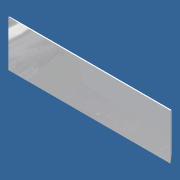
# Autodesk Inventor part: bottom panel right
Saved by Autodesk Inventor 2012 (Build 160160000, 160)
## iProperties
Created: 2012-02-06
Part Number: bottom panel right
Material: Default
Document SubType Name: Modeling
Designer: Allison Garza
Density: 1 g/cm^3
Author: Allison Garza
Autodesk Inventor part; units mm, degrees
ref_plane "YZ Plane" through (0, 0, 0) normal (1, 0, 0) x (0, 1, 0)
ref_plane "XZ Plane" through (0, 0, 0) normal (0, 1, 0) x (-1, 0, 0)
ref_plane "XY Plane" through (0, 0, 0) normal (0, 0, 1) x (1, 0, 0)
sketch "Sketch1" plane through (0, 0, 0) normal (0, 0, 1) x (1, 0, 0)
  line L0 (-37.1429, 20.9244) -> (432.7571, 20.9244)
  line L1 (432.7571, 20.9244) -> (432.7571, -112.4256)
  line L2 (432.7571, -112.4256) -> (-37.1429, -112.4256)
  line L3 (-37.1429, -112.4256) -> (-37.1429, 20.9244)
  point P0 (0, 0)
  dimension "d0" = 469.9
  dimension "d1" = 133.35
  constraints: 8 end point, 2 parallel, 1 horizontal, 1 perpendicular
  measures "d0" distance of L0.start L0.end
  measures "d1" distance of L2.end L0.start
extrude "Extrusion1" add sketch "Sketch1" along normal blind 3.175
sketch "Sketch2" plane through (432.7571, -112.4256, 0) normal (1, 0, 0) x (0, 0, -1)
  line L0 (0, 133.35) -> (0, 0) projected
  line L1 (-3.175, 133.35) -> (0, 107.95)
  line L2 (-3.175, 0) -> (0, 22.86)
  line L3 (-3.175, 0) -> (0, 0)
  line L4 (0, 22.86) -> (0, 0)
  point P0 (0, 112.4256)
  dimension "d4" = 25.4
  dimension "d5" = 22.86
  constraints: 8 end point, 2 perpendicular, 2 point on line
  measures "d4" vertical distance of L1.start L1.end
  measures "d5" vertical distance of L2.end L2.start
extrude "Extrusion3" cut sketch "Sketch2" against normal blind 476.25
body "Solid1"
